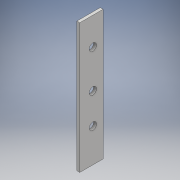
# Autodesk Inventor part: Gear wall motor side
Saved by Autodesk Inventor 2017 (Build 210142000, 142)
## iProperties
Created: 2017-11-21
Part Number: Gear wall motor side
Material: Generic
Document SubType Name: Modeling
Designer: Shlomee
Density: 1 g/cm^3
Appearance: Default
Author: Shlomee
Autodesk Inventor part; units mm, degrees
ref_plane "YZ Plane" through (0, 0, 0) normal (1, 0, 0) x (0, 1, 0)
ref_plane "XZ Plane" through (0, 0, 0) normal (0, 1, 0) x (-1, 0, 0)
ref_plane "XY Plane" through (0, 0, 0) normal (0, 0, 1) x (1, 0, 0)
sketch "Sketch1" plane through (0, 0, 0) normal (0, 0, 1) x (1, 0, 0)
  line L0 (-1.1274, 1.6306) -> (0.8726, 1.6306)
  line L1 (0.8726, 1.6306) -> (0.8726, -14.3694)
  line L2 (0.8726, -14.3694) -> (-1.1274, -14.3694)
  line L3 (-1.1274, -14.3694) -> (-1.1274, 1.6306)
  point P0 (0, 0)
  dimension "d0" = 2
  dimension "d1" = 16
  constraints: 8 end point, 2 parallel, 1 horizontal, 1 perpendicular
  measures "d0" distance of L0.start L0.end
  measures "d1" distance of L0.end L1.end
extrude "Extrusion1" add sketch "Sketch1" along normal blind 89
sketch "Sketch2" plane through (0.8726, -14.3694, 0) normal (1, 0, 0) x (0, 0, -1)
  circle A0 centre (-23.0575, 8.9801) radius 2.5 projected
  circle A1 centre (-23.0575, 8.9801) radius 2.5 projected
  circle A2 centre (-23.0575, 8.9801) radius 2.5 projected
  circle A3 centre (-44.0219, 8.9592) radius 2.5 projected
  circle A4 centre (-44.0219, 8.9592) radius 2.5 projected
  circle A5 centre (-44.0219, 8.9592) radius 2.5 projected
  circle A6 centre (-44.0219, 8.9592) radius 2.5 projected
  circle A7 centre (-44.0219, 8.9592) radius 2.5 projected
  circle A8 centre (-70.0331, 8.9359) radius 2.5 projected
  point P0 (0, 14.3694)
extrude "Extrusion2" cut sketch "Sketch2" against normal blind 10
body "Solid1"
